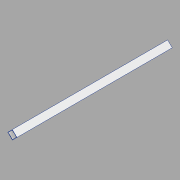
# Autodesk Inventor part: base_rail
Saved by Autodesk Inventor 2020 (Build 240168000, 168)
## iProperties
Created: 2021-04-01
Part Number: base_rail
Material: Aluminum 6061
Document SubType Name: Modeling
Designer: griss
Density: 2.7 g/cm^3
Appearance: Aluminum - Flat
Author: griss
Autodesk Inventor part; units mm, degrees
ref_plane "YZ Plane" through (0, 0, 0) normal (1, 0, 0) x (0, 1, 0)
ref_plane "XZ Plane" through (0, 0, 0) normal (0, 1, 0) x (-1, 0, 0)
ref_plane "XY Plane" through (0, 0, 0) normal (0, 0, 1) x (1, 0, 0)
sketch "Sketch1" plane through (0, 0, 0) normal (0, 0, 1) x (1, 0, 0)
  line L0 (0, 17.9605) -> (17.9605, 0)
  line L1 (17.9605, 0) -> (0, -17.9605)
  line L2 (0, -17.9605) -> (-17.9605, 0)
  line L3 (-17.9605, 0) -> (0, 17.9605)
  line L4 (0, 17.9605) -> (0, -17.9605) construction
  line L5 (17.9605, 0) -> (-17.9605, 0) construction
  point P0 (0, 0)
  point P1 (0, 0)
  point P2 (0, 0)
  point P3 (0, 0)
  dimension "d2" = 25.4
  dimension "d3" = 25.4
  constraints: 12 end point, 4 midpoint, 2 parallel, 1 coincident, 1 horizontal alignment, 1 perpendicular
  measures "d2" distance of L1.end L2.end
  measures "d3" distance of L0.end L1.end
extrude "Extrusion1" add sketch "Sketch1" along normal mid plane 609.6
shell "Shell1" thickness 1.27 removed faces 2 at (0, -5.9868, 304.8) at (0, -5.9868, -304.8)
body "Solid1"
